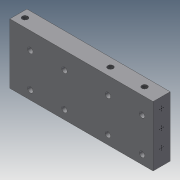
# Autodesk Inventor part: XGuideBracket
Saved by Autodesk Inventor 2019 (Build 230136000, 136)
## iProperties
Created: 2018-10-20
Part Number: XGuideBracket
Material: Generic
Document SubType Name: Modeling
Designer: LillaHunden
Density: 1 g/cm^3
Appearance: Default
Mass: 16.35 g
Surface Area: 76.85 cm^2
Volume: 16.35 cm^3
Author: LillaHunden
Autodesk Inventor part; units mm, degrees
ref_plane "YZ Plane" through (0, 0, 0) normal (1, 0, 0) x (0, 1, 0)
ref_plane "XZ Plane" through (0, 0, 0) normal (0, 1, 0) x (-1, 0, 0)
ref_plane "XY Plane" through (0, 0, 0) normal (0, 0, 1) x (1, 0, 0)
sketch "Sketch1" plane through (0, 0, 0) normal (0, 0, 1) x (1, 0, 0)
  line L0 (30.8973, 7.322) -> (-53.1027, 7.322)
  line L1 (-53.1027, 7.322) -> (-53.1027, -32.678)
  line L2 (-53.1027, -32.678) -> (30.8973, -32.678)
  line L3 (30.8973, -32.678) -> (30.8973, 7.322)
  dimension "d2" = 84
  dimension "d3" = 40
  constraints: 8 end point, 2 parallel, 1 horizontal, 1 perpendicular
  measures "d2" distance of L2.end L1.end
  measures "d3" distance of L1.end L0.end
extrude "Extrusion1" add sketch "Sketch1" along normal blind 10
sketch "Sketch3" plane through (0, 0, 0) normal (0, 0, -1) x (-1, 0, 0)
  point P0 (-24.3973, -2.678)
  point P1 (-4.3973, -2.678)
  point P2 (-4.3973, -22.678)
  point P3 (-24.3973, -22.678)
  point P4 (21.1027, -2.678)
  point P5 (41.1027, -2.678)
  point P6 (41.1027, -22.678)
  point P7 (21.1027, -22.678)
hole "Hole1" at (24.3973, -2.678, 0) at (4.3973, -2.678, 0) at (4.3973, -22.678, 0) at (24.3973, -22.678, 0) at (-21.1027, -2.678, 0) at (-41.1027, -2.678, 0) at (-41.1027, -22.678, 0) at (-21.1027, -22.678, 0) direction (0, 0, 1) diameter 3.2 depth 10 counterbore diameter 6.7 counterbore depth 3.6
sketch "Sketch4" plane through (-53.1027, 7.322, 0) normal (0, 1, 0) x (1, 0, 0)
  point P0 (74, -5)
  point P1 (54, -5)
  point P2 (7.9048, -5)
hole "Hole3" at (20.8973, 7.322, 5) at (0.8973, 7.322, 5) at (-45.1979, 7.322, 5) direction (0, -1, 0) diameter 3.242 depth 8.6 tip angle 120 thread size "M4x0.7" class "6H" standard "ISO Metric profile"
sketch "Sketch8" plane through (-53.1027, -32.678, 0) normal (0, -1, 0) x (1, 0, 0)
  line L0 (0, 0) -> (84, 0) projected
  line L1 (84, 0) -> (84, 10) projected
  line L2 (0, 10) -> (84, 10) projected
  line L3 (0, 0) -> (0, 10) projected
  point P0 (53.1027, 0)
extrude "Extrusion2" cut sketch "Sketch8" against normal blind 4.75
sketch "Sketch7" plane through (30.8973, -32.678, 0) normal (1, 0, 0) x (0, 0, -1)
  point P0 (-5, 14)
  point P1 (-5, 24)
  point P2 (-5, 34)
sketch "Sketch9" plane through (30.8973, 7.322, 10) normal (1, 0, 0) x (0, 0, -1)
  point P0 (5, -6)
  point P1 (5, -26)
  point P2 (5, -16)
hole "Hole8" at (30.8973, 1.322, 5) at (30.8973, -18.678, 5) at (30.8973, -8.678, 5) direction (-1, 0, 0) diameter 3 depth 6.3506 tip angle 120
chamfer "Chamfer1" distance 1.5 angle 45 1 edges at (-11.1027, -27.928, 0)
body "Solid1"
